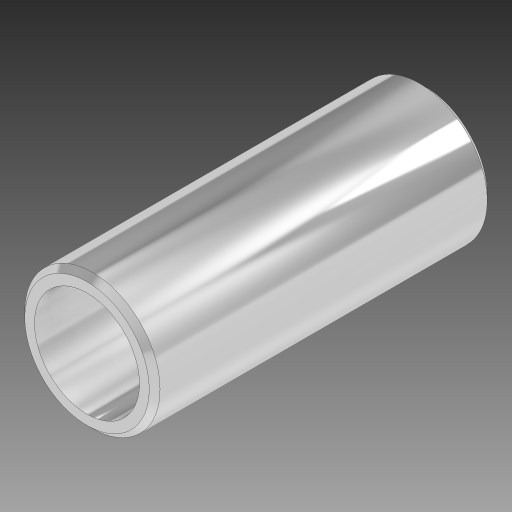
# Autodesk Inventor part: Elevator Cascade Pulley Bearing Spacer
Saved by Autodesk Inventor 2024 (Build 280153000, 153)
## iProperties
Created: 2023-05-06
Part Number: Elevator Cascade Pulley Bearing Spacer
Material: Aluminum
Document SubType Name: Modeling
Designer: Max Boord
Mass: 0.536633 g
Surface Area: 5.81538 cm^2
Volume: 0.198753 cm^3
Density: 2.7 g/cm^3
Appearance: Chrome - Polished
Author: Max Boord
Autodesk Inventor part; units mm, degrees
ref_plane "YZ Plane" through (0, 0, 0) normal (1, 0, 0) x (0, 1, 0)
ref_plane "XZ Plane" through (0, 0, 0) normal (0, 1, 0) x (-1, 0, 0)
ref_plane "XY Plane" through (0, 0, 0) normal (0, 0, 1) x (1, 0, 0)
sketch "Sketch1" plane through (0, 0, 0) normal (0, 0, 1) x (1, 0, 0)
  circle A0 centre (0, 0) radius 3.175
  dimension "d0" = 6.35
  constraints: 1 centre point, 1 coincident
  measures "d0" diameter of A0
extrude "Extrusion1" add sketch "Sketch1" along normal mid plane 15.875
sketch "Sketch2" plane through (0, 0, 7.9375) normal (0, 0, 1) x (1, 0, 0)
  circle A0 centre (0, 0) radius 3.175 projected
  constraints: 1 coincident
hole "Hole1" at (0, 0, 7.9375) direction (0, 0, -1) diameter 4.9276 end through all
chamfer "Chamfer1" distance 0.254 angle 45 2 edges at (-3.175, 0, 7.9375) (-3.175, 0, -7.9375)
body "Solid1"
